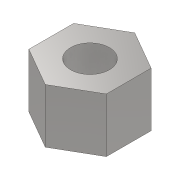
# Autodesk Inventor part: M2_nut
Saved by Autodesk Inventor 2022 (Build 260153000, 153)
## iProperties
Created: 2022-10-11
Part Number: M2_nut
Material: Generic
Document SubType Name: Modeling
Designer: dell
Density: 1 g/cm^3
Appearance: Stainless - Brushed
Author: dell
Autodesk Inventor part; units mm, degrees
ref_plane "YZ Plane" through (0, 0, 0) normal (1, 0, 0) x (0, 1, 0)
ref_plane "XZ Plane" through (0, 0, 0) normal (0, 1, 0) x (-1, 0, 0)
ref_plane "XY Plane" through (0, 0, 0) normal (0, 0, 1) x (1, 0, 0)
sketch "Sketch1" plane through (0, 0, 0) normal (0, 1, 0) x (-1, 0, 0)
  line L0 (0, -2.3094) -> (-2, -1.1547)
  line L1 (-2, -1.1547) -> (-2, 1.1547)
  line L2 (-2, 1.1547) -> (0, 2.3094)
  line L3 (0, 2.3094) -> (2, 1.1547)
  line L4 (2, 1.1547) -> (2, -1.1547)
  line L5 (2, -1.1547) -> (0, -2.3094)
  circle A0 centre (0, 0) radius 1
  dimension "d0" = 4
  dimension "d1" = 2
  constraints: 12 end point, 2 coincident, 1 centre point, 13 other
  measures "d0" distance between parallel lines of L1 L4
  measures "d1" diameter of A0
extrude "Extrusion1" add sketch "Sketch1" along normal blind 2.8
body "Solid1"
